Autodesk Inventor part; units mm, degrees
(part 2 of 2)
sketch "Sketch18" plane through (0, 0, 0) normal (0, 0, 1) x (1, 0, 0)
  circle A0 centre (6.1, 11.9) radius 0.15 projected
  circle A1 centre (6.1, 13.5) radius 0.15 projected
  circle A2 centre (22.375, -7.815) radius 0.15 projected
  circle A3 centre (39.71, -9.9) radius 0.15 projected
  circle A4 centre (48.4, -3.8) radius 0.15 projected
  circle A5 centre (55.95, 2.9) radius 0.15 projected
  circle A6 centre (79, 24.8) radius 0.15 projected
  circle A7 centre (52.3, 16.9) radius 0.15 projected
  circle A8 centre (36, 1.1) radius 0.15 projected
  circle A9 centre (83.5, -20.09) radius 0.15 projected
  circle A10 centre (80.4, -15.3) radius 0.15 projected
  circle A11 centre (36.4, -40.4) radius 0.15 projected
  circle A12 centre (17.7, -11.2) radius 0.15 projected
  circle A13 centre (20.6, -14.5) radius 0.15 projected
  circle A14 centre (6.475, -9) radius 0.15 projected
  circle A15 centre (81.1, -6.7) radius 0.15 projected
  circle A16 centre (81.1, -12.3) radius 0.15 projected
  circle A17 centre (67.69, 14.95) radius 0.15 projected
  circle A18 centre (42.638, 24.252) radius 0.15 projected
  circle A19 centre (71.9, 18.8) radius 0.15 projected
  circle A20 centre (42.73, 22.395) radius 0.15 projected
  circle A21 centre (55.56, 27.69) radius 0.15 projected
  circle A22 centre (70.1, 24.7) radius 0.15 projected
  circle A23 centre (82, 18.7) radius 0.15 projected
  circle A24 centre (30.03, 31.595) radius 0.15 projected
  circle A25 centre (29.2, 18.3) radius 0.15 projected
  circle A26 centre (83.6, -26) radius 0.15 projected
  circle A27 centre (83.5, -21.8) radius 0.15 projected
  circle A28 centre (89.2, -12.4) radius 0.15 projected
  circle A29 centre (59.9, -31.6) radius 0.15 projected
  circle A30 centre (36.075, -13.17) radius 0.15 projected
  circle A31 centre (20, -37.1) radius 0.15 projected
  circle A32 centre (9.7, -43.3) radius 0.15 projected
  circle A33 centre (31.7, -33.7) radius 0.15 projected
  circle A34 centre (34.4, -38) radius 0.15 projected
  circle A35 centre (30.5, -43.4) radius 0.15 projected
  circle A36 centre (28.255, -10.955) radius 0.15 projected
  circle A37 centre (28.525, 3.19) radius 0.15 projected
  circle A38 centre (71.4, -31.6) radius 0.15 projected
  circle A39 centre (38.76, -24.905) radius 0.15 projected
  circle A40 centre (64.22, 34.51) radius 0.15 projected
  circle A41 centre (18.46, -4.74) radius 0.15 projected
  circle A42 centre (50.28, 18.42) radius 0.15 projected
  circle A43 centre (22, -40) radius 0.15 projected
  circle A44 centre (27.195, -8.84) radius 0.15 projected
  circle A45 centre (38.3, 36) radius 0.15 projected
  circle A46 centre (74.66, -17.095) radius 0.15 projected
  circle A47 centre (56.99, 5.41) radius 0.15 projected
  circle A48 centre (81.9, 22.5) radius 0.15 projected
  circle A49 centre (25.955, -10.94) radius 0.15 projected
  circle A50 centre (12.3, -10.2) radius 0.15 projected
  circle A51 centre (29.44, -12.665) radius 0.15 projected
  circle A52 centre (26.715, -10.94) radius 0.15 projected
  circle A53 centre (12.3, -9.4) radius 0.15 projected
  circle A54 centre (35.36, -13.43) radius 0.15 projected
  circle A55 centre (26.94, -34.355) radius 0.15 projected
  circle A56 centre (74.56, -18.975) radius 0.15 projected
  circle A57 centre (72.38, 10.4) radius 0.15 projected
  circle A58 centre (28.44, -32.03) radius 0.15 projected
  circle A59 centre (27.66, -34.62) radius 0.15 projected
  circle A60 centre (77.1, -17.9) radius 0.15 projected
  circle A61 centre (76.33, 18.885) radius 0.15 projected
  circle A62 centre (77.1, -18.7) radius 0.15 projected
  circle A63 centre (76.87, 18.35) radius 0.15 projected
  circle A64 centre (27.195, -9.92) radius 0.15 projected
  circle A65 centre (54.885, -4.415) radius 0.15 projected
  circle A66 centre (58.69, -20.96) radius 0.15 projected
  circle A67 centre (30.62, -26.105) radius 0.15 projected
  circle A68 centre (51.44, 19.365) radius 0.15 projected
  circle A69 centre (36.14, 18.41) radius 0.15 projected
  circle A70 centre (58, -20.64) radius 0.15 projected
  circle A71 centre (31.34, -25.84) radius 0.15 projected
  circle A72 centre (50.95, 18.78) radius 0.15 projected
  circle A73 centre (35.36, 18.425) radius 0.15 projected
  circle A74 centre (5.9, -7.5) radius 0.15 projected
  circle A75 centre (27.6, -14.51) radius 0.15 projected
  circle A76 centre (5.9, -10.5) radius 0.15 projected
  circle A77 centre (5.9, -9.5) radius 0.15 projected
  circle A78 centre (18.2, -16.5) radius 0.15 projected
  circle A79 centre (11.9, -15.4) radius 0.15 projected
  circle A80 centre (39.69, 0.21) radius 0.15 projected
  circle A81 centre (30.03, 30.83) radius 0.15 projected
  circle A82 centre (62.6, 19.84) radius 0.15 projected
  circle A83 centre (68.7, 10.4) radius 0.15 projected
  circle A84 centre (48.485, 0.89) radius 0.15 projected
  circle A85 centre (55.7, -14.5) radius 0.15 projected
  circle A86 centre (31.58, -16.8) radius 0.15 projected
  circle A87 centre (60.54, 5.13) radius 0.15 projected
  circle A88 centre (46.6, 2.4) radius 0.15 projected
  circle A89 centre (5.9, 14.5) radius 0.15 projected
  circle A90 centre (27.9, 4.7) radius 0.15 projected
  circle A91 centre (30.67, 6.93) radius 0.15 projected
  circle A92 centre (5.9, 16.5) radius 0.15 projected
  circle A93 centre (27.9, 8.7) radius 0.15 projected
  circle A94 centre (30.67, 8.36) radius 0.15 projected
  circle A95 centre (28.96, 10.535) radius 0.15 projected
  circle A96 centre (5.9, 18.5) radius 0.15 projected
  circle A97 centre (25.9, 15.1) radius 0.15 projected
  circle A98 centre (5.9, 20.5) radius 0.15 projected
  circle A99 centre (27.9, 16.7) radius 0.15 projected
  circle A100 centre (63.455, -20.64) radius 0.15 projected
  circle A101 centre (28.315, -9.36) radius 0.15 projected
  circle A102 centre (18.44, -2.79) radius 0.15 projected
  circle A103 centre (34.67, 7.705) radius 0.15 projected
  circle A104 centre (25.9, 32.7) radius 0.15 projected
  circle A105 centre (29.9, 18) radius 0.15 projected
  circle A106 centre (26.9, 19.2) radius 0.15 projected
  circle A107 centre (27.89, 20.7) radius 0.15 projected
  circle A108 centre (27.8, 23.1) radius 0.15 projected
  circle A109 centre (27.9, 24.7) radius 0.15 projected
  circle A110 centre (28.095, 26.88) radius 0.15 projected
  circle A111 centre (27.9, 28.7) radius 0.15 projected
  circle A112 centre (25.8, 31.1) radius 0.15 projected
  circle A113 centre (25.8, 35.1) radius 0.15 projected
  circle A114 centre (25.9, 36.7) radius 0.15 projected
  circle A115 centre (25.8, 39.1) radius 0.15 projected
  circle A116 centre (27.615, 38.87) radius 0.15 projected
  circle A117 centre (28.03, 40.835) radius 0.15 projected
  circle A118 centre (9.1, 22.5) radius 0.15 projected
  circle A119 centre (9.3, 25.5) radius 0.15 projected
  circle A120 centre (5.9, 26.5) radius 0.15 projected
  circle A121 centre (5.9, 28.5) radius 0.15 projected
  circle A122 centre (5.9, 30.5) radius 0.15 projected
  circle A123 centre (5.9, 32.5) radius 0.15 projected
  circle A124 centre (5.9, 33.5) radius 0.15 projected
  circle A125 centre (5.9, 34.5) radius 0.15 projected
  circle A126 centre (9.55, -9.34) radius 0.15 projected
  circle A127 centre (17.6, -37.7) radius 0.15 projected
  circle A128 centre (30.815, -16.8) radius 0.15 projected
  circle A129 centre (32.1, -44.4) radius 0.15 projected
  circle A130 centre (72.8, 16.2) radius 0.15 projected
  circle A131 centre (30, 39.4) radius 0.15 projected
  circle A132 centre (42.9, -27.9) radius 0.15 projected
  circle A133 centre (45.3, -23.4) radius 0.15 projected
  circle A134 centre (44.5, -24.2) radius 0.15 projected
  circle A135 centre (44.5, -22.6) radius 0.15 projected
  circle A136 centre (19.3, -0.5) radius 0.15 projected
  circle A137 centre (18.5, 0.3) radius 0.15 projected
  circle A138 centre (20.1, 0.3) radius 0.15 projected
  circle A139 centre (19.3, 1.1) radius 0.15 projected
  circle A140 centre (88, -34.7) radius 0.15 projected
  circle A141 centre (43.7, -23.4) radius 0.15 projected
  circle A142 centre (42.3, -22.9) radius 0.15 projected
  circle A143 centre (13, 44.4) radius 0.15 projected
  circle A144 centre (21.8, 36.5) radius 0.15 projected
  circle A145 centre (23.8, 28.5) radius 0.15 projected
  circle A146 centre (23.815, 20.5) radius 0.15 projected
  circle A147 centre (16, 22.5) radius 0.15 projected
  circle A148 centre (14, 30.5) radius 0.15 projected
  circle A149 centre (14, 38.5) radius 0.15 projected
  circle A150 centre (89.2, -34.7) radius 0.15 projected
  circle A151 centre (49.9, -10.235) radius 0.15 projected
  circle A152 centre (38.9, 2.5) radius 0.15 projected
  circle A153 centre (44.92, 10.98) radius 0.15 projected
  circle A154 centre (58.69, 28.175) radius 0.15 projected
  circle A155 centre (37.5, 41.6) radius 0.15 projected
  circle A156 centre (36.7, 43.2) radius 0.15 projected
  circle A157 centre (37.5, 42.4) radius 0.15 projected
  circle A158 centre (21.8, 42) radius 0.15 projected
  circle A159 centre (21.8, 34) radius 0.15 projected
  circle A160 centre (23.9, 22) radius 0.15 projected
  circle A161 centre (16, 23.98) radius 0.15 projected
  circle A162 centre (14.005, 31.98) radius 0.15 projected
  circle A163 centre (14.005, 39.975) radius 0.15 projected
  circle A164 centre (41.7, 39.2) radius 0.15 projected
  circle A165 centre (39.69, -0.55) radius 0.15 projected
  circle A166 centre (79.6, 11.8) radius 0.15 projected
  circle A167 centre (85.6, 12.1) radius 0.15 projected
  circle A168 centre (89.4, -31.4) radius 0.15 projected
  circle A169 centre (17, -12.91) radius 0.15 projected
  circle A170 centre (15.4, -11) radius 0.15 projected
  circle A171 centre (88.2, -12.7) radius 0.15 projected
  circle A172 centre (86.4, -28.8) radius 0.15 projected
  circle A173 centre (81.5, -31.5) radius 0.15 projected
  circle A174 centre (88.4, 13) radius 0.15 projected
  circle A175 centre (85.6, -29.1) radius 0.15 projected
  circle A176 centre (85.2, 28.9) radius 0.15 projected
  circle A177 centre (83, -24.1) radius 0.15 projected
  circle A178 centre (50.4, 11.1) radius 0.15 projected
  circle A179 centre (71.28, -18.24) radius 0.15 projected
  circle A180 centre (61, 18.735) radius 0.15 projected
  circle A181 centre (75.1, 17.3) radius 0.15 projected
  circle A182 centre (46.3, 19.8) radius 0.15 projected
  circle A183 centre (52.5, 14.6) radius 0.15 projected
  circle A184 centre (44.1, 22.1) radius 0.15 projected
  circle A185 centre (36.2, -35.4) radius 0.15 projected
  circle A186 centre (20.9, -41.7) radius 0.15 projected
  circle A187 centre (83.9, -17.2) radius 0.15 projected
  circle A188 centre (34.9, -39.7) radius 0.15 projected
  circle A189 centre (56.315, 27.375) radius 0.15 projected
  circle A190 centre (6.8, -39.2) radius 0.15 projected
  circle A191 centre (73.9, 28.4) radius 0.15 projected
  circle A192 centre (48.3, 26.6) radius 0.15 projected
  circle A193 centre (48.3, 25) radius 0.15 projected
  circle A194 centre (46.7, 25) radius 0.15 projected
  circle A195 centre (23.9, 18) radius 0.15 projected
  circle A196 centre (23.8, 10) radius 0.15 projected
  circle A197 centre (16, 7.98) radius 0.15 projected
  circle A198 centre (16, 15.98) radius 0.15 projected
  circle A199 centre (11.795, 7.67) radius 0.15 projected
  circle A200 centre (52.3, -42.3) radius 0.15 projected
  circle A201 centre (4.3, -36.6) radius 0.15 projected
  circle A202 centre (61, 12.46) radius 0.15 projected
  circle A203 centre (81.5, -26.1) radius 0.15 projected
  circle A204 centre (61.1, -29) radius 0.15 projected
  circle A205 centre (61.9, -29) radius 0.15 projected
  circle A206 centre (62.8, -29.8) radius 0.15 projected
  circle A207 centre (55, -41.1) radius 0.15 projected
  circle A208 centre (55, -40.3) radius 0.15 projected
  circle A209 centre (53, -41.5) radius 0.15 projected
  circle A210 centre (27.1, 15.2) radius 0.15 projected
  circle A211 centre (23.8, 12.5) radius 0.15 projected
  circle A212 centre (23.8, 4.5) radius 0.15 projected
  circle A213 centre (16, 10.5) radius 0.15 projected
  circle A214 centre (20.7, -36.8) radius 0.15 projected
  circle A215 centre (55.96, 26.7) radius 0.15 projected
  circle A216 centre (28.4, -18.5) radius 0.15 projected
  circle A217 centre (44.5, -14.6) radius 0.15 projected
  circle A218 centre (50.3, 2) radius 0.15 projected
  circle A219 centre (46.1, -10.8) radius 0.15 projected
  circle A220 centre (51.395, 20.445) radius 0.15 projected
  circle A221 centre (77.6, 23.5) radius 0.15 projected
  circle A222 centre (36.1, 2.8) radius 0.15 projected
  circle A223 centre (61.465, -22.4) radius 0.15 projected
  circle A224 centre (80.3, -11.5) radius 0.15 projected
  circle A225 centre (80.1, -35.8) radius 0.15 projected
  circle A226 centre (29.2, -42.7) radius 0.15 projected
  circle A227 centre (36.025, 15.595) radius 0.15 projected
  circle A228 centre (29.8, 34.1) radius 0.15 projected
  circle A229 centre (22.4, -12.1) radius 0.15 projected
  circle A230 centre (8.09, -8.99) radius 0.15 projected
  circle A231 centre (72.62, -11.01) radius 0.15 projected
  circle A232 centre (66.42, 15.715) radius 0.15 projected
  circle A233 centre (53.89, -5.83) radius 0.15 projected
  circle A234 centre (72.94, -11.7) radius 0.15 projected
  circle A235 centre (69.5, 19.215) radius 0.15 projected
  circle A236 centre (71.76, -12.19) radius 0.15 projected
  circle A237 centre (65.88, 16.255) radius 0.15 projected
  circle A238 centre (53.71, -6.57) radius 0.15 projected
  circle A239 centre (58.84, -22.08) radius 0.15 projected
  circle A240 centre (67.3, 19.215) radius 0.15 projected
  circle A241 centre (81.7, -33.4) radius 0.15 projected
  circle A242 centre (5.3, -38.3) radius 0.15 projected
  circle A243 centre (83.355, -3.96) radius 0.15 projected
  circle A244 centre (84.5, 13.8) radius 0.15 projected
  circle A245 centre (82.7, -14.2) radius 0.15 projected
  circle A246 centre (83.5, -14.2) radius 0.15 projected
  circle A247 centre (83.5, -15) radius 0.15 projected
  circle A248 centre (82.7, -15.8) radius 0.15 projected
  circle A249 centre (66.3, -36.73) radius 0.15 projected
  circle A250 centre (68.5, 37.65) radius 0.15 projected
  circle A251 centre (70.2, -37.9) radius 0.15 projected
  circle A252 centre (37.8, -35.6) radius 0.15 projected
  circle A253 centre (38.7, -41.5) radius 0.15 projected
  circle A254 centre (38.7, -35.5) radius 0.15 projected
  circle A255 centre (72, 27.6) radius 0.15 projected
  circle A256 centre (71.18, 27.71) radius 0.15 projected
  circle A257 centre (69, 28.1) radius 0.15 projected
  circle A258 centre (56.4, 36.81) radius 0.15 projected
  circle A259 centre (81.5, 14.6) radius 0.15 projected
  circle A260 centre (82.1, 15.2) radius 0.15 projected
  circle A261 centre (81.8, 17.59) radius 0.15 projected
  circle A262 centre (81.2, 16.99) radius 0.15 projected
  circle A263 centre (81.5, 15.2) radius 0.15 projected
  circle A264 centre (62.8, -39.2) radius 0.15 projected
  circle A265 centre (71.39, -36.73) radius 0.15 projected
  circle A266 centre (62, 39.1) radius 0.15 projected
  circle A267 centre (70, 28.3) radius 0.15 projected
  circle A268 centre (69.9, -2.2) radius 0.15 projected
  circle A269 centre (81.78, -23.295) radius 0.15 projected
  circle A270 centre (72.04, -18.24) radius 0.15 projected
  circle A271 centre (71.4, -7.4) radius 0.15 projected
  circle A272 centre (87.095, 35.64) radius 0.15 projected
  circle A273 centre (72.76, -19.96) radius 0.15 projected
  circle A274 centre (85.155, -30.25) radius 0.15 projected
  circle A275 centre (77.34, 13.12) radius 0.15 projected
  circle A276 centre (78.29, -34.2) radius 0.15 projected
  circle A277 centre (6.1, 6.3) radius 0.15 projected
  circle A278 centre (6.1, 7.9) radius 0.15 projected
  circle A279 centre (6.1, 9.5) radius 0.15 projected
  circle A280 centre (6.1, 11.1) radius 0.15 projected
  circle A281 centre (41, -36.2) radius 0.15 projected
  circle A282 centre (45.6, 19.5) radius 0.15 projected
  circle A283 centre (35.7, -24.95) radius 0.15 projected
  circle A284 centre (82, 13.8) radius 0.15 projected
  circle A285 centre (83.2, 10.9) radius 0.15 projected
  circle A286 centre (43.2, 20.1) radius 0.15 projected
  circle A287 centre (77.9, 41.2) radius 0.15 projected
  circle A288 centre (89.4, -37.7) radius 0.15 projected
  circle A289 centre (59.1, -32.9) radius 0.15 projected
  circle A290 centre (79.8, -31.7) radius 0.15 projected
  circle A291 centre (12, -41.3) radius 0.15 projected
  circle A292 centre (70.1, -34.7) radius 0.15 projected
  circle A293 centre (68.2, -38.9) radius 0.15 projected
  circle A294 centre (73.8, -42.9) radius 0.15 projected
  circle A295 centre (64.8, -42.9) radius 0.15 projected
  circle A296 centre (53.1, -31.5) radius 0.15 projected
  circle A297 centre (52.6, -28) radius 0.15 projected
  circle A298 centre (51.8, -28.8) radius 0.15 projected
  circle A299 centre (50.2, -28.8) radius 0.15 projected
  circle A300 centre (42.4, -37.1) radius 0.15 projected
  circle A301 centre (42.4, -35.4) radius 0.15 projected
  circle A302 centre (42.2, -39.8) radius 0.15 projected
  circle A303 centre (41, -39.8) radius 0.15 projected
  circle A304 centre (41, -37.8) radius 0.15 projected
  circle A305 centre (42.2, -37.8) radius 0.15 projected
  circle A306 centre (47.4, -43) radius 0.15 projected
  circle A307 centre (47.4, -44.4) radius 0.15 projected
  circle A308 centre (46.6, -43.1) radius 0.15 projected
  circle A309 centre (35.3, 27.2) radius 0.15 projected
  circle A310 centre (29.47, 15.2) radius 0.15 projected
  circle A311 centre (22, 18.695) radius 0.15 projected
  circle A312 centre (69.7, 29.7) radius 0.15 projected
  circle A313 centre (64.2, 32.9) radius 0.15 projected
  circle A314 centre (73.5, 33) radius 0.15 projected
  circle A315 centre (68.2, 36.7) radius 0.15 projected
  circle A316 centre (61.95, 43.2) radius 0.15 projected
  circle A317 centre (57.2, 38.9) radius 0.15 projected
  circle A318 centre (40.5, 30) radius 0.15 projected
  circle A319 centre (44, 19.5) radius 0.15 projected
  circle A320 centre (43.2, 20.7) radius 0.15 projected
  circle A321 centre (39.8, 35.2) radius 0.15 projected
  circle A322 centre (39.8, 36.4) radius 0.15 projected
  circle A323 centre (41.8, 36.4) radius 0.15 projected
  circle A324 centre (41.8, 35.2) radius 0.15 projected
  circle A325 centre (39.7, 31.6) radius 0.15 projected
  circle A326 centre (36.9, 39.6) radius 0.15 projected
  circle A327 centre (35.2, 38.8) radius 0.15 projected
  circle A328 centre (35.2, 40.4) radius 0.15 projected
  circle A329 centre (51.4, 42.2) radius 0.15 projected
  circle A330 centre (51.4, 43.8) radius 0.15 projected
  circle A331 centre (52.5, 35.9) radius 0.15 projected
  circle A332 centre (12.8, -10.8) radius 0.15 projected
  circle A333 centre (21.7, 39.7) radius 0.15 projected
  circle A334 centre (21.69, 31.695) radius 0.15 projected
  circle A335 centre (23.7, 23.7) radius 0.15 projected
  circle A336 centre (23.7, 15.7) radius 0.15 projected
  circle A337 centre (23.7, 7.7) radius 0.15 projected
  circle A338 centre (15.9, 5.7) radius 0.15 projected
  circle A339 centre (15.9, 13.7) radius 0.15 projected
  circle A340 centre (16, 21.7) radius 0.15 projected
  circle A341 centre (13.9, 29.7) radius 0.15 projected
  circle A342 centre (13.9, 41.7) radius 0.15 projected
  circle A343 centre (13.9, 37.7) radius 0.15 projected
  circle A344 centre (13.9, 33.7) radius 0.15 projected
  circle A345 centre (16, 25.7) radius 0.15 projected
  circle A346 centre (16, 17.7) radius 0.15 projected
  circle A347 centre (16, 9.7) radius 0.15 projected
  circle A348 centre (23.7, 3.7) radius 0.15 projected
  circle A349 centre (23.915, 11.745) radius 0.15 projected
  circle A350 centre (23.765, 19.74) radius 0.15 projected
  circle A351 centre (23.7, 27.7) radius 0.15 projected
  circle A352 centre (21.7, 35.7) radius 0.15 projected
  circle A353 centre (10.29, 10.02) radius 0.15 projected
  circle A354 centre (37.7, 36.5) radius 0.15 projected
  circle A355 centre (51.3, 31.8) radius 0.15 projected
  circle A356 centre (51.4, 43) radius 0.15 projected
  circle A357 centre (52.2, 42.2) radius 0.15 projected
  circle A358 centre (35.2, 39.6) radius 0.15 projected
  circle A359 centre (36.9, 40.4) radius 0.15 projected
  circle A360 centre (36.9, 38.8) radius 0.15 projected
  circle A361 centre (39.7, 30.8) radius 0.15 projected
  circle A362 centre (42.1, 35.8) radius 0.15 projected
  circle A363 centre (40.8, 36.5) radius 0.15 projected
  circle A364 centre (39.5, 35.8) radius 0.15 projected
  circle A365 centre (43.2, 19.5) radius 0.15 projected
  circle A366 centre (44.8, 19.5) radius 0.15 projected
  circle A367 centre (40.5, 31.6) radius 0.15 projected
  circle A368 centre (57.2, 36) radius 0.15 projected
  circle A369 centre (64.8, 40.7) radius 0.15 projected
  circle A370 centre (59.3, 30.1) radius 0.15 projected
  circle A371 centre (71, 36.7) radius 0.15 projected
  circle A372 centre (63.6, 30.8) radius 0.15 projected
  circle A373 centre (66.6, 31.9) radius 0.15 projected
  circle A374 centre (10.6, 42) radius 0.15 projected
  circle A375 centre (22, 9.7) radius 0.15 projected
  circle A376 centre (40, 22.6) radius 0.15 projected
  circle A377 centre (39.4, 27.1) radius 0.15 projected
  circle A378 centre (46.6, -44.4) radius 0.15 projected
  circle A379 centre (47.4, -43.7) radius 0.15 projected
  circle A380 centre (46.6, -43.7) radius 0.15 projected
  circle A381 centre (41.6, -37.8) radius 0.15 projected
  circle A382 centre (40.9, -38.8) radius 0.15 projected
  circle A383 centre (41.6, -40.1) radius 0.15 projected
  circle A384 centre (41.6, -35.4) radius 0.15 projected
  circle A385 centre (43.2, -35.4) radius 0.15 projected
  circle A386 centre (41.7, -37.1) radius 0.15 projected
  circle A387 centre (51, -28.8) radius 0.15 projected
  circle A388 centre (52.6, -28.8) radius 0.15 projected
  circle A389 centre (52.6, -27.2) radius 0.15 projected
  circle A390 centre (57.6, -40) radius 0.15 projected
  circle A391 centre (64.7, -39.8) radius 0.15 projected
  circle A392 centre (73.5, -40.62) radius 0.15 projected
  circle A393 centre (64.7, -34.7) radius 0.15 projected
  circle A394 centre (60, -34.6) radius 0.15 projected
  circle A395 centre (6.7, -40.65) radius 0.15 projected
  circle A396 centre (84.6, -33) radius 0.15 projected
  circle A397 centre (82.75, -5.8) radius 0.15 projected
  circle A398 centre (54, 33) radius 0.15 projected
  circle A399 centre (77.7, 35) radius 0.15 projected
  circle A400 centre (45.6, 20.1) radius 0.15 projected
  circle A401 centre (78.415, 10.635) radius 0.15 projected
  circle A402 centre (58, 1.5) radius 0.15 projected
  circle A403 centre (38.2, -15.4) radius 0.15 projected
  circle A404 centre (52.2, 43) radius 0.15 projected
  circle A405 centre (41, -37) radius 0.15 projected
  circle A406 centre (6.1, 10.3) radius 0.15 projected
  circle A407 centre (6.1, 8.7) radius 0.15 projected
  circle A408 centre (6.1, 7.1) radius 0.15 projected
  circle A409 centre (6.1, 5.5) radius 0.15 projected
  circle A410 centre (87.1, 36.4) radius 0.15 projected
  circle A411 centre (71.66, -8.115) radius 0.15 projected
  circle A412 centre (72.8, -18.24) radius 0.15 projected
  circle A413 centre (78.29, -35) radius 0.15 projected
  circle A414 centre (77.335, 13.88) radius 0.15 projected
  circle A415 centre (85.155, -31.015) radius 0.15 projected
  circle A416 centre (72, -19.96) radius 0.15 projected
  circle A417 centre (66, -2.185) radius 0.15 projected
  circle A418 centre (56.6, 33.9) radius 0.15 projected
  circle A419 centre (68.4, 33.9) radius 0.15 projected
  circle A420 centre (60.9, 32.5) radius 0.15 projected
  circle A421 centre (62.5, -35.8) radius 0.15 projected
  circle A422 centre (67.1, -32.9) radius 0.15 projected
  circle A423 centre (81.8, 16.99) radius 0.15 projected
  circle A424 centre (80.6, 16.99) radius 0.15 projected
  circle A425 centre (81.2, 17.59) radius 0.15 projected
  circle A426 centre (82.1, 14.6) radius 0.15 projected
  circle A427 centre (68.2, 2) radius 0.15 projected
  circle A428 centre (62, 33.1) radius 0.15 projected
  circle A429 centre (74.5, 37.3) radius 0.15 projected
  circle A430 centre (72.5, 34.9) radius 0.15 projected
  circle A431 centre (58, -36.75) radius 0.15 projected
  circle A432 centre (59.1, -39.8) radius 0.15 projected
  circle A433 centre (75, -37.9) radius 0.15 projected
  circle A434 centre (75.5, -41.6) radius 0.15 projected
  circle A435 centre (37.86, -38.715) radius 0.15 projected
  circle A436 centre (66.3, -43.2) radius 0.15 projected
  circle A437 centre (84.3, -15) radius 0.15 projected
  circle A438 centre (83.5, -15.8) radius 0.15 projected
  circle A439 centre (84.3, -14.2) radius 0.15 projected
  circle A440 centre (82.7, -15) radius 0.15 projected
  circle A441 centre (65.6, 33.5) radius 0.15 projected
  circle A442 centre (70.7, -4.8) radius 0.15 projected
  circle A443 centre (77, 37.5) radius 0.15 projected
  circle A444 centre (18.7, -43.7) radius 0.15 projected
  circle A445 centre (87.2, -34.6) radius 0.15 projected
  circle A446 centre (65.34, 16.795) radius 0.15 projected
  circle A447 centre (71.54, -11.46) radius 0.15 projected
  circle A448 centre (68, 18.915) radius 0.15 projected
  circle A449 centre (58.08, -22.08) radius 0.15 projected
  circle A450 centre (54.345, -6.99) radius 0.15 projected
  circle A451 centre (66.96, 15.175) radius 0.15 projected
  circle A452 centre (59.17, -23.16) radius 0.15 projected
  circle A453 centre (68.8, 18.915) radius 0.15 projected
  circle A454 centre (59.93, -23.17) radius 0.15 projected
  circle A455 centre (54.57, -5.49) radius 0.15 projected
  circle A456 centre (6.2, -11.2) radius 0.15 projected
  circle A457 centre (22.4, -15) radius 0.15 projected
  circle A458 centre (34.9, 32.9) radius 0.15 projected
  circle A459 centre (28.5, -39.9) radius 0.15 projected
  circle A460 centre (13.9, -44) radius 0.15 projected
  circle A461 centre (77.395, -37.24) radius 0.15 projected
  circle A462 centre (78.1, -11.1) radius 0.15 projected
  circle A463 centre (47.7, 6.3) radius 0.15 projected
  circle A464 centre (22.6, -0.4) radius 0.15 projected
  circle A465 centre (63.7, 13.27) radius 0.15 projected
  circle A466 centre (44.8, 13.3) radius 0.15 projected
  circle A467 centre (38.1, -9.9) radius 0.15 projected
  circle A468 centre (61.82, -4.17) radius 0.15 projected
  circle A469 centre (24.9, -17.7) radius 0.15 projected
  circle A470 centre (64.69, 33.91) radius 0.15 projected
  circle A471 centre (39.3, -25.44) radius 0.15 projected
  circle A472 centre (16, 14.5) radius 0.15 projected
  circle A473 centre (16, 6.5) radius 0.15 projected
  circle A474 centre (23.8, 8.5) radius 0.15 projected
  circle A475 centre (23.8, 16.5) radius 0.15 projected
  circle A476 centre (52.3, -41.5) radius 0.15 projected
  circle A477 centre (53, -42.3) radius 0.15 projected
  circle A478 centre (55.8, -40.3) radius 0.15 projected
  circle A479 centre (62.8, -29) radius 0.15 projected
  circle A480 centre (61.9, -29.8) radius 0.15 projected
  circle A481 centre (61.9, -28.2) radius 0.15 projected
  circle A482 centre (61.1, -28.2) radius 0.15 projected
  circle A483 centre (81.2, 25.9) radius 0.15 projected
  circle A484 centre (51.3, -13.2) radius 0.15 projected
  circle A485 centre (61.1, -29.8) radius 0.15 projected
  circle A486 centre (53.8, -42.3) radius 0.15 projected
  circle A487 centre (12.3, 7.1) radius 0.15 projected
  circle A488 centre (15.995, 11.98) radius 0.15 projected
  circle A489 centre (23.8, 6) radius 0.15 projected
  circle A490 centre (23.8, 14) radius 0.15 projected
  circle A491 centre (45.9, 25) radius 0.15 projected
  circle A492 centre (47.5, 25) radius 0.15 projected
  circle A493 centre (48.3, 25.8) radius 0.15 projected
  circle A494 centre (82, -4.3) radius 0.15 projected
  circle A495 centre (64.22, 18.4) radius 0.15 projected
  circle A496 centre (13.7, 4.4) radius 0.15 projected
  circle A497 centre (40.7, -42.7) radius 0.15 projected
  circle A498 centre (83.9, -22.5) radius 0.15 projected
  circle A499 centre (82.4, -25.6) radius 0.15 projected
  circle A500 centre (24, -42.8) radius 0.15 projected
  circle A501 centre (81.9, 23.3) radius 0.15 projected
  circle A502 centre (54.4, 15.9) radius 0.15 projected
  circle A503 centre (26.7, -4.3) radius 0.15 projected
  circle A504 centre (71.18, 17.96) radius 0.15 projected
  circle A505 centre (71.66, 12.95) radius 0.15 projected
  circle A506 centre (65.465, 13.585) radius 0.15 projected
  circle A507 centre (36, 4.7) radius 0.15 projected
  circle A508 centre (89.8, 14.2) radius 0.15 projected
  circle A509 centre (82.2, -24.1) radius 0.15 projected
  circle A510 centre (84.4, 28.9) radius 0.15 projected
  circle A511 centre (88.6, 28.4) radius 0.15 projected
  circle A512 centre (81, 31.3) radius 0.15 projected
  circle A513 centre (87.2, -28.8) radius 0.15 projected
  circle A514 centre (88.3, -31.1) radius 0.15 projected
  circle A515 centre (87.4, -12.7) radius 0.15 projected
  circle A516 centre (15.4, -12.6) radius 0.15 projected
  circle A517 centre (15.45, -35.315) radius 0.15 projected
  circle A518 centre (87.3, 12.1) radius 0.15 projected
  circle A519 centre (69.8, 2.8) radius 0.15 projected
  circle A520 centre (5.9, -5.5) radius 0.15 projected
  circle A521 centre (78.82, 13.46) radius 0.15 projected
  circle A522 centre (14, 44) radius 0.15 projected
  circle A523 centre (14, 35.98) radius 0.15 projected
  circle A524 centre (16.005, 27.98) radius 0.15 projected
  circle A525 centre (16, 19.98) radius 0.15 projected
  circle A526 centre (23.8, 26) radius 0.15 projected
  circle A527 centre (21.8, 38) radius 0.15 projected
  circle A528 centre (23.58, 30.6) radius 0.15 projected
  circle A529 centre (36.7, 42.4) radius 0.15 projected
  circle A530 centre (37.5, 43.2) radius 0.15 projected
  circle A531 centre (36.7, 41.6) radius 0.15 projected
  circle A532 centre (48.935, 19.86) radius 0.15 projected
  circle A533 centre (57.11, -21.28) radius 0.15 projected
  circle A534 centre (38.9, 4.2) radius 0.15 projected
  circle A535 centre (83, -37) radius 0.15 projected
  circle A536 centre (14, 42.5) radius 0.15 projected
  circle A537 centre (14, 34.5) radius 0.15 projected
  circle A538 centre (16, 26.5) radius 0.15 projected
  circle A539 centre (16, 18.5) radius 0.15 projected
  circle A540 centre (23.8, 24.5) radius 0.15 projected
  circle A541 centre (21.765, 32.54) radius 0.15 projected
  circle A542 centre (21.8, 40.5) radius 0.15 projected
  circle A543 centre (42.9, -22.6) radius 0.15 projected
  circle A544 centre (43.7, -22.6) radius 0.15 projected
  circle A545 centre (43.7, -24.2) radius 0.15 projected
  circle A546 centre (18.5, 1.1) radius 0.15 projected
  circle A547 centre (20.1, 1.1) radius 0.15 projected
  circle A548 centre (19.3, 0.3) radius 0.15 projected
  circle A549 centre (18.5, -0.5) radius 0.15 projected
  circle A550 centre (42.295, -15.04) radius 0.15 projected
  circle A551 centre (44.5, -23.4) radius 0.15 projected
  circle A552 centre (45.3, -24.2) radius 0.15 projected
  circle A553 centre (45.3, -22.6) radius 0.15 projected
  circle A554 centre (39.9, -33.9) radius 0.15 projected
  circle A555 centre (74.765, 16.16) radius 0.15 projected
  circle A556 centre (39.2, -44) radius 0.15 projected
  circle A557 centre (28.855, -9.895) radius 0.15 projected
  circle A558 centre (39.98, -26.8) radius 0.15 projected
  circle A559 centre (5.9, 35.5) radius 0.15 projected
  circle A560 centre (10.1, -6.5) radius 0.15 projected
  circle A561 centre (12.1, 40.835) radius 0.15 projected
  circle A562 centre (11.7, 39.45) radius 0.15 projected
  circle A563 centre (5.9, 31.5) radius 0.15 projected
  circle A564 centre (5.9, 29.5) radius 0.15 projected
  circle A565 centre (5.9, 27.5) radius 0.15 projected
  circle A566 centre (5.9, 25.6) radius 0.15 projected
  circle A567 centre (5.9, 22.4) radius 0.15 projected
  circle A568 centre (5.9, 21.5) radius 0.15 projected
  circle A569 centre (33.84, 20.76) radius 0.15 projected
  circle A570 centre (33.67, 20.015) radius 0.15 projected
  circle A571 centre (32.76, 20.76) radius 0.15 projected
  circle A572 centre (32, 20.76) radius 0.15 projected
  circle A573 centre (31.87, 20.01) radius 0.15 projected
  circle A574 centre (32.37, 17.98) radius 0.15 projected
  circle A575 centre (32.19, 15.57) radius 0.15 projected
  circle A576 centre (32.49, 14.87) radius 0.15 projected
  circle A577 centre (32.01, 14.28) radius 0.15 projected
  circle A578 centre (33.8, 9.5) radius 0.15 projected
  circle A579 centre (30.03, 12.85) radius 0.15 projected
  circle A580 centre (33.165, 9.08) radius 0.15 projected
  circle A581 centre (41.53, 21.79) radius 0.15 projected
  circle A582 centre (31.87, 19.245) radius 0.15 projected
  circle A583 centre (29.71, 3.92) radius 0.15 projected
  circle A584 centre (20.29, -10.94) radius 0.15 projected
  circle A585 centre (31.88, -25.3) radius 0.15 projected
  circle A586 centre (46.1, -6.8) radius 0.15 projected
  circle A587 centre (29.71, 11.64) radius 0.15 projected
  circle A588 centre (5.9, 19.5) radius 0.15 projected
  circle A589 centre (29.68, 10.88) radius 0.15 projected
  circle A590 centre (27.89, 12.5) radius 0.15 projected
  circle A591 centre (28.2, 10.6) radius 0.15 projected
  circle A592 centre (34.8, -43.4) radius 0.15 projected
  circle A593 centre (30.93, 7.645) radius 0.15 projected
  circle A594 centre (27.8, 7.3) radius 0.15 projected
  circle A595 centre (5.9, 15.5) radius 0.15 projected
  circle A596 centre (45.85, 4.725) radius 0.15 projected
  circle A597 centre (60, 3.5) radius 0.15 projected
  circle A598 centre (31.03, 2.045) radius 0.15 projected
  circle A599 centre (29.395, -9.36) radius 0.15 projected
  circle A600 centre (55.7, -15.63) radius 0.15 projected
  circle A601 centre (81.79, 24.055) radius 0.15 projected
  circle A602 centre (66.69, 5.48) radius 0.15 projected
  circle A603 centre (81.9, 26.3) radius 0.15 projected
  circle A604 centre (28.7, 39.8) radius 0.15 projected
  circle A605 centre (40.01, 0.9) radius 0.15 projected
  circle A606 centre (41.41, 0.69) radius 0.15 projected
  circle A607 centre (18.7, -10.605) radius 0.15 projected
  circle A608 centre (18.7, -14.1) radius 0.15 projected
  circle A609 centre (5.9, -8.5) radius 0.15 projected
  circle A610 centre (41.09, 0) radius 0.15 projected
  circle A611 centre (24.875, -10.94) radius 0.15 projected
  circle A612 centre (33.9, 32.1) radius 0.15 projected
  circle A613 centre (15.01, -42.2) radius 0.15 projected
  circle A614 centre (19.26, -3.56) radius 0.15 projected
  circle A615 centre (51.675, -11.495) radius 0.15 projected
  circle A616 centre (34.66, 32.175) radius 0.15 projected
  circle A617 centre (15.21, -43.025) radius 0.15 projected
  circle A618 centre (19.525, -4.275) radius 0.15 projected
  circle A619 centre (52.215, -10.96) radius 0.15 projected
  circle A620 centre (48.5, -1.81) radius 0.15 projected
  circle A621 centre (12.3, -7.8) radius 0.15 projected
  circle A622 centre (28.285, -14.12) radius 0.15 projected
  circle A623 centre (71.62, 10.405) radius 0.15 projected
  circle A624 centre (74.02, -18.435) radius 0.15 projected
  circle A625 centre (71.62, 9.63) radius 0.15 projected
  circle A626 centre (73.48, -17.9) radius 0.15 projected
  circle A627 centre (28.44, -33.87) radius 0.15 projected
  circle A628 centre (77.41, 18.885) radius 0.15 projected
  circle A629 centre (77.1, -19.5) radius 0.15 projected
  circle A630 centre (28.12, -33.18) radius 0.15 projected
  circle A631 centre (50.5, 7.1) radius 0.15 projected
  circle A632 centre (16.1, -35.72) radius 0.15 projected
  circle A633 centre (28.9, -13.205) radius 0.15 projected
  circle A634 centre (12.3, -8.6) radius 0.15 projected
  circle A635 centre (27.475, -10.94) radius 0.15 projected
  circle A636 centre (29.44, -13.745) radius 0.15 projected
  circle A637 centre (36.65, -41.35) radius 0.15 projected
  circle A638 centre (77.95, 18.35) radius 0.15 projected
  circle A639 centre (5.9, 17.5) radius 0.15 projected
  circle A640 centre (48.4, -3) radius 0.15 projected
  circle A641 centre (40.95, 23.5) radius 0.15 projected
  circle A642 centre (57.3, 13.8) radius 0.15 projected
  circle A643 centre (61.67, 19.095) radius 0.15 projected
  circle A644 centre (25.2, -38.3) radius 0.15 projected
  circle A645 centre (14.2, -34.58) radius 0.15 projected
  circle A646 centre (56.72, 26.73) radius 0.15 projected
  circle A647 centre (14.96, -35.9) radius 0.15 projected
  circle A648 centre (63.735, -31.04) radius 0.15 projected
  circle A649 centre (40.1, -20.565) radius 0.15 projected
  circle A650 centre (87.7, -33.2) radius 0.15 projected
  circle A651 centre (40.7, -44) radius 0.15 projected
  circle A652 centre (34.5, -35.8) radius 0.15 projected
  circle A653 centre (22.1, -43.9) radius 0.15 projected
  circle A654 centre (39.66, -26.11) radius 0.15 projected
  circle A655 centre (18.72, -5.455) radius 0.15 projected
  circle A656 centre (70.6, -31.6) radius 0.15 projected
  circle A657 centre (86, -12.4) radius 0.15 projected
  circle A658 centre (78.9, -21.3) radius 0.15 projected
  circle A659 centre (81.4, -22.6) radius 0.15 projected
  circle A660 centre (84.8, -29.1) radius 0.15 projected
  circle A661 centre (29.2, 39.2) radius 0.15 projected
  circle A662 centre (63.68, 35.415) radius 0.15 projected
  circle A663 centre (78.71, 18.4) radius 0.15 projected
  circle A664 centre (73, 21.9) radius 0.15 projected
  circle A665 centre (57.5, 16) radius 0.15 projected
  circle A666 centre (29.6, -4.4) radius 0.15 projected
  circle A667 centre (71.79, 13.7) radius 0.15 projected
  circle A668 centre (55.9, 13.9) radius 0.15 projected
  circle A669 centre (88.44, 15.85) radius 0.15 projected
  circle A670 centre (78.18, -10.195) radius 0.15 projected
  circle A671 centre (71.46, -20.495) radius 0.15 projected
  circle A672 centre (6.475, -7) radius 0.15 projected
  circle A673 centre (20.6, -17.3) radius 0.15 projected
  circle A674 centre (31.1, 33.25) radius 0.15 projected
  circle A675 centre (29.4, -39.5) radius 0.15 projected
  circle A676 centre (80.1, -33.8) radius 0.15 projected
  circle A677 centre (46.9, 6.3) radius 0.15 projected
  circle A678 centre (23.9, -1.6) radius 0.15 projected
  circle A679 centre (37.1, 16.6) radius 0.15 projected
  circle A680 centre (21.1, -42.5) radius 0.15 projected
  circle A681 centre (57, -2.2) radius 0.15 projected
  circle A682 centre (47.5, -10.8) radius 0.15 projected
  circle A683 centre (54, 5.6) radius 0.15 projected
  circle A684 centre (53.9, 1) radius 0.15 projected
  circle A685 centre (6.1, 12.7) radius 0.15 projected
  circle A686 centre (82.985, -17.14) radius 0.15 projected
  circle A687 centre (58.9, -42.5) radius 0.175 projected
  circle A688 centre (37.4, -31.2) radius 0.175 projected
  circle A689 centre (35.8, -29.6) radius 0.175 projected
  circle A690 centre (57.3, 44.1) radius 0.175 projected
  circle A691 centre (38.531, 28.469) radius 0.175 projected
  circle A692 centre (56.169, 41.369) radius 0.175 projected
  circle A693 centre (56.169, 43.631) radius 0.175 projected
  circle A694 centre (58.431, 43.631) radius 0.175 projected
  circle A695 centre (88.531, -4.369) radius 0.175 projected
  circle A696 centre (37.4, 28) radius 0.175 projected
  circle A697 centre (35.8, 29.6) radius 0.175 projected
  circle A698 centre (37.4, 31.2) radius 0.175 projected
  circle A699 centre (39, 29.6) radius 0.175 projected
  circle A700 centre (88.531, -6.631) radius 0.175 projected
  circle A701 centre (86.269, -6.631) radius 0.175 projected
  circle A702 centre (86.269, -4.369) radius 0.175 projected
  circle A703 centre (77.031, 4.369) radius 0.175 projected
  circle A704 centre (74.769, 4.369) radius 0.175 projected
  circle A705 centre (74.769, 6.631) radius 0.175 projected
  circle A706 centre (77.031, 6.631) radius 0.175 projected
  circle A707 centre (58.431, -43.631) radius 0.175 projected
  circle A708 centre (56.169, -43.631) radius 0.175 projected
  circle A709 centre (56.169, -41.369) radius 0.175 projected
  circle A710 centre (58.431, -41.369) radius 0.175 projected
  circle A711 centre (57.3, -40.9) radius 0.175 projected
  circle A712 centre (55.7, -42.5) radius 0.175 projected
  circle A713 centre (57.3, -44.1) radius 0.175 projected
  circle A714 centre (77.5, 5.5) radius 0.175 projected
  circle A715 centre (75.9, 7.1) radius 0.175 projected
  circle A716 centre (74.3, 5.5) radius 0.175 projected
  circle A717 centre (75.9, 3.9) radius 0.175 projected
  circle A718 centre (87.4, -3.9) radius 0.175 projected
  circle A719 centre (85.8, -5.5) radius 0.175 projected
  circle A720 centre (87.4, -7.1) radius 0.175 projected
  circle A721 centre (89, -5.5) radius 0.175 projected
  circle A722 centre (38.531, 30.731) radius 0.175 projected
  circle A723 centre (36.269, 30.731) radius 0.175 projected
  circle A724 centre (36.269, 28.469) radius 0.175 projected
  circle A725 centre (39, -29.6) radius 0.175 projected
  circle A726 centre (58.9, 42.5) radius 0.175 projected
  circle A727 centre (38.531, -28.469) radius 0.175 projected
  circle A728 centre (55.7, 42.5) radius 0.175 projected
  circle A729 centre (57.3, 40.9) radius 0.175 projected
  circle A730 centre (37.4, -28) radius 0.175 projected
  circle A731 centre (36.269, -28.469) radius 0.175 projected
  circle A732 centre (36.269, -30.731) radius 0.175 projected
  circle A733 centre (38.531, -30.731) radius 0.175 projected
  circle A734 centre (58.431, 41.369) radius 0.175 projected
  circle A735 centre (34.1, 39.2) radius 0.35 projected
  circle A736 centre (87.975, 4.15) radius 0.35 projected
  circle A737 centre (80.725, 4.15) radius 0.35 projected
  circle A738 centre (36.1, -33.4) radius 0.35 projected
  circle A739 centre (7.9, 9.6) radius 0.5 projected
  circle A740 centre (12.3, -3.9) radius 0.5 projected
  circle A741 centre (62.54, -8) radius 0.6 projected
  circle A742 centre (62.54, 8) radius 0.6 projected
  circle A743 centre (57.46, 8) radius 0.6 projected
  circle A744 centre (57.46, -8) radius 0.6 projected
  circle A745 centre (37.4, 29.6) radius 1.1 projected
  circle A746 centre (87.4, -5.5) radius 1.1 projected
  circle A747 centre (37.4, -29.6) radius 1.1 projected
  circle A748 centre (57.3, -42.5) radius 1.1 projected
  circle A749 centre (75.9, 5.5) radius 1.1 projected
  circle A750 centre (57.3, 42.5) radius 1.1 projected
  circle A751 centre (32.5, -11.5) radius 1.5 projected
  circle A752 centre (32.5, 11.5) radius 1.5 projected
  circle A753 centre (76, 30.5) radius 1.5 projected
  circle A754 centre (76, -30.5) radius 1.5 projected
  circle A755 centre (32.5, 30.5) radius 1.5 projected
  circle A756 centre (76, 11.5) radius 1.5 projected
  circle A757 centre (76, -11.5) radius 1.5 projected
  circle A758 centre (32.5, -30.5) radius 1.5 projected
  arc A759 (90.4, 34) -> (89.4, 35) centre (89.4, 34) ccw projected
  arc A760 (88.4, 36) -> (89.4, 35) centre (89.4, 36) ccw projected
  line L0 (88.4, 36) -> (88.4, 42) projected
  arc A761 (89.4, 43) -> (88.4, 42) centre (89.4, 42) ccw projected
  arc A762 (89.4, 43) -> (90.4, 44) centre (89.4, 44) ccw projected
  line L1 (90.4, 44) -> (90.4, 47.4) projected
  arc A763 (90.4, 47.4) -> (89.9, 47.9) centre (89.9, 47.4) ccw projected
  line L2 (89.9, 47.9) -> (10.5, 47.9) projected
  arc A764 (10.5, 47.9) -> (10, 47.4) centre (10.5, 47.4) ccw projected
  line L3 (10, 47.4) -> (10, 36.65) projected
  arc A765 (9.5, 36.15) -> (10, 36.65) centre (9.5, 36.65) ccw projected
  line L4 (9.5, 36.15) -> (0.5, 36.15) projected
  line L5 (0, 35.65) -> (0.5, 36.15) projected
  line L6 (0, 35.65) -> (0, 25.45) projected
  line L7 (0.5, 24.95) -> (0, 25.45) projected
  line L8 (0.5, 24.95) -> (8.4, 24.95) projected
  arc A766 (8.4, 23.05) -> (8.4, 24.95) centre (8.4, 24) ccw projected
  line L9 (8.4, 23.05) -> (0.5, 23.05) projected
  line L10 (0, 22.55) -> (0.5, 23.05) projected
  line L11 (0, 22.55) -> (0, -14.65) projected
  line L12 (0.5, -15.15) -> (0, -14.65) projected
  line L13 (0.5, -15.15) -> (10, -15.15) projected
  arc A767 (10, -18.65) -> (10, -15.15) centre (10, -16.9) ccw projected
  line L14 (10, -18.65) -> (2.5, -18.65) projected
  arc A768 (2.5, -18.65) -> (2, -19.15) centre (2.5, -19.15) ccw projected
  line L15 (2, -19.15) -> (2, -47.4) projected
  arc A769 (2, -47.4) -> (2.5, -47.9) centre (2.5, -47.4) ccw projected
  line L16 (2.5, -47.9) -> (89.9, -47.9) projected
  arc A770 (89.9, -47.9) -> (90.4, -47.4) centre (89.9, -47.4) ccw projected
  line L17 (90.4, -47.4) -> (90.4, -4) projected
  arc A771 (90.4, -4) -> (89.4, -3) centre (89.4, -4) ccw projected
  line L18 (89.4, -3) -> (75.9, -3) projected
  arc A772 (74.9, -2) -> (75.9, -3) centre (75.9, -2) ccw projected
  line L19 (74.9, -2) -> (74.9, 2) projected
  arc A773 (75.9, 3) -> (74.9, 2) centre (75.9, 2) ccw projected
  line L20 (75.9, 3) -> (89.4, 3) projected
  arc A774 (89.4, 3) -> (90.4, 4) centre (89.4, 4) ccw projected
  line L21 (90.4, 4) -> (90.4, 34) projected
  point P0 (0, 0)
  point P1 (1.5, -42.9)
  point P2 (9.5, 37.9)
  point P3 (9.5, 38.9)
  point P4 (1.5, -41.9)
  point P5 (9.5, 39.9)
  point P6 (1.5, -40.9)
  point P7 (9.5, 40.9)
  point P8 (1.5, -39.9)
  point P9 (9.5, 41.9)
  point P10 (1.5, -38.9)
  point P11 (9.5, 42.9)
  point P12 (1.5, -37.9)
  point P13 (9.5, 43.9)
  point P14 (1.5, -36.9)
  point P15 (8.5, 37.9)
  point P16 (0.5, -42.9)
  point P17 (8.5, 38.9)
  point P18 (0.5, -41.9)
  point P19 (8.5, 39.9)
  point P20 (0.5, -40.9)
  point P21 (8.5, 40.9)
  point P22 (0.5, -39.9)
  point P23 (8.5, 41.9)
  point P24 (0.5, -38.9)
  point P25 (8.5, 42.9)
  point P26 (0.5, -37.9)
  point P27 (8.5, 43.9)
  point P28 (0.5, -36.9)
  point P29 (7.5, 37.9)
  point P30 (-0.5, -42.9)
  point P31 (7.5, 38.9)
  point P32 (-0.5, -41.9)
  point P33 (7.5, 39.9)
  point P34 (-0.5, -40.9)
  point P35 (7.5, 40.9)
  point P36 (-0.5, -39.9)
  point P37 (7.5, 41.9)
  point P38 (-0.5, -38.9)
  point P39 (7.5, 42.9)
  point P40 (-0.5, -37.9)
  point P41 (7.5, 43.9)
  point P42 (-0.5, -36.9)
  point P43 (6.5, 37.9)
  point P44 (-1.5, -42.9)
  point P45 (6.5, 38.9)
  point P46 (-1.5, -41.9)
  point P47 (6.5, 39.9)
  point P48 (-1.5, -40.9)
  point P49 (6.5, 40.9)
  point P50 (-1.5, -39.9)
  point P51 (6.5, 41.9)
  point P52 (-1.5, -38.9)
  point P53 (6.5, 42.9)
  point P54 (-1.5, -37.9)
  point P55 (6.5, 43.9)
  point P56 (-1.5, -36.9)
  dimension "d159" = 0.5
  dimension "d161" = 5
  dimension "d162" = 0.5
  dimension "d163" = 10
  dimension "d166" = 1
  dimension "d169" = 1
  constraints: 1 horizontal, 1 vertical, 54 other
  measures "d159" distance from line of L15 point (1.5, -42.9)
  measures "d161" distance from line of point (1.5, -42.9) L16
  measures "d162" distance from line of point (9.5, 37.9) L3
  measures "d163" distance from line of point (9.5, 37.9) L2
  measures "d166" distance of point (9.5, 37.9) point (9.5, 38.9)
  measures "d169" distance of point (9.5, 37.9) point (8.5, 37.9)
ref_plane "Work Plane1" through (16, 0, 0) normal (1, 0, 0) x (0, 1, 0)
sketch "Sketch19" plane through (16, 0, 0) normal (1, 0, 0) x (0, 1, 0)
  line L0 (-4, -0.8) -> (-4, 0.8) projected
  line L1 (-47.4, 0.8) -> (-4, 0.8) projected
  line L2 (-47.4, -0.8) -> (-47.4, 0.8) projected
  line L3 (-4, -0.8) -> (-47.4, -0.8) projected
  point P0 (0, 0)
  point P1 (-42.9, 1.8)
  point P2 (37.9, 1.8)
  point P3 (-42.9, 0)
  point P4 (37.9, 0)
  point P5 (-42.9, 2.8)
  point P6 (37.9, 2.8)
  point P7 (-41.9, 1.8)
  point P8 (38.9, 1.8)
  point P9 (-41.9, 2.8)
  point P10 (38.9, 2.8)
  point P11 (-40.9, 1.8)
  point P12 (39.9, 1.8)
  point P13 (-40.9, 2.8)
  point P14 (39.9, 2.8)
  point P15 (-39.9, 1.8)
  point P16 (40.9, 1.8)
  point P17 (-39.9, 2.8)
  point P18 (40.9, 2.8)
  point P19 (-38.9, 1.8)
  point P20 (41.9, 1.8)
  point P21 (-38.9, 2.8)
  point P22 (41.9, 2.8)
  point P23 (-37.9, 1.8)
  point P24 (42.9, 1.8)
  point P25 (-37.9, 2.8)
  point P26 (42.9, 2.8)
  point P27 (-36.9, 1.8)
  point P28 (43.9, 1.8)
  point P29 (-36.9, 2.8)
  point P30 (43.9, 2.8)
  point P31 (-42.9, 3.8)
  point P32 (37.9, 3.8)
  point P33 (-41.9, 3.8)
  point P34 (38.9, 3.8)
  point P35 (-40.9, 3.8)
  point P36 (39.9, 3.8)
  point P37 (-39.9, 3.8)
  point P38 (40.9, 3.8)
  point P39 (-38.9, 3.8)
  point P40 (41.9, 3.8)
  point P41 (-37.9, 3.8)
  point P42 (42.9, 3.8)
  point P43 (-36.9, 3.8)
  point P44 (43.9, 3.8)
  point P45 (-42.9, 4.8)
  point P46 (37.9, 4.8)
  point P47 (-41.9, 4.8)
  point P48 (38.9, 4.8)
  point P49 (-40.9, 4.8)
  point P50 (39.9, 4.8)
  point P51 (-39.9, 4.8)
  point P52 (40.9, 4.8)
  point P53 (-38.9, 4.8)
  point P54 (41.9, 4.8)
  point P55 (-37.9, 4.8)
  point P56 (42.9, 4.8)
  point P57 (-36.9, 4.8)
  point P58 (43.9, 4.8)
  point P59 (-42.9, 5.8)
  point P60 (37.9, 5.8)
  point P61 (-41.9, 5.8)
  point P62 (38.9, 5.8)
  point P63 (-40.9, 5.8)
  point P64 (39.9, 5.8)
  point P65 (-39.9, 5.8)
  point P66 (40.9, 5.8)
  point P67 (-38.9, 5.8)
  point P68 (41.9, 5.8)
  point P69 (-37.9, 5.8)
  point P70 (42.9, 5.8)
  point P71 (-36.9, 5.8)
  point P72 (43.9, 5.8)
  point P73 (-42.9, 6.8)
  point P74 (37.9, 6.8)
  point P75 (-41.9, 6.8)
  point P76 (38.9, 6.8)
  point P77 (-40.9, 6.8)
  point P78 (39.9, 6.8)
  point P79 (-39.9, 6.8)
  point P80 (40.9, 6.8)
  point P81 (-38.9, 6.8)
  point P82 (41.9, 6.8)
  point P83 (-37.9, 6.8)
  point P84 (42.9, 6.8)
  point P85 (-36.9, 6.8)
  point P86 (43.9, 6.8)
  point P87 (-42.9, 7.8)
  point P88 (37.9, 7.8)
  point P89 (-41.9, 7.8)
  point P90 (38.9, 7.8)
  point P91 (-40.9, 7.8)
  point P92 (39.9, 7.8)
  point P93 (-39.9, 7.8)
  point P94 (40.9, 7.8)
  point P95 (-38.9, 7.8)
  point P96 (41.9, 7.8)
  point P97 (-37.9, 7.8)
  point P98 (42.9, 7.8)
  point P99 (-36.9, 7.8)
  point P100 (43.9, 7.8)
  dimension "d175" = 1
  dimension "d178" = 1
  dimension "d181" = 1
  constraints: 2 vertical alignment, 1 horizontal, 1 horizontal alignment, 1 vertical, 96 other
  measures "d175" distance of point (-42.9, 1.8) point (-42.9, 2.8)
  measures "d178" distance of point (-42.9, 1.8) point (-41.9, 1.8)
  measures "d181" distance from line of L1 point (-42.9, 1.8)
ref_plane "Work Plane2" through (41, 0, 0) normal (1, 0, 0) x (0, 1, 0)
sketch "Sketch20" plane through (41, 0, 0) normal (1, 0, 0) x (0, 1, 0)
  point P0 (0, 0)
  point P1 (-42.9, 1.8)
  point P2 (-42.9, 2.8)
  point P3 (-41.9, 2.8)
  point P4 (-41.9, 1.8)
  point P5 (-40.9, 1.8)
  point P6 (-40.9, 2.8)
  point P7 (-39.9, 2.8)
  point P8 (-39.9, 1.8)
  point P9 (-38.9, 1.8)
  point P10 (-38.9, 2.8)
  point P11 (-37.9, 1.8)
  point P12 (-37.9, 2.8)
  point P13 (-36.9, 2.8)
  point P14 (-36.9, 1.8)
  point P15 (37.9, 1.8)
  point P16 (38.9, 1.8)
  point P17 (39.9, 1.8)
  point P18 (40.9, 1.8)
  point P19 (41.9, 1.8)
  point P20 (42.9, 1.8)
  point P21 (43.9, 1.8)
  point P22 (43.9, 2.8)
  point P23 (42.9, 2.8)
  point P24 (41.9, 2.8)
  point P25 (40.9, 2.8)
  point P26 (39.9, 2.8)
  point P27 (38.9, 2.8)
  point P28 (37.9, 2.8)
  point P29 (-42.9, 3.8)
  point P30 (-41.9, 3.8)
  point P31 (-40.9, 3.8)
  point P32 (-39.9, 3.8)
ref_plane "Work Plane3" through (4, 0, 0) normal (1, 0, 0) x (0, 1, 0)
sketch "Sketch21" plane through (4, 0, 0) normal (1, 0, 0) x (0, 1, 0)
  point P0 (0, 0)
  point P1 (-42.9, 3.8)
  point P2 (-41.9, 3.8)
  point P3 (-40.9, 3.8)
  point P4 (-39.9, 3.8)
  point P5 (-38.9, 3.8)
  point P6 (-37.9, 3.8)
  point P7 (-36.9, 3.8)
  point P8 (-36.9, 4.8)
  point P9 (-37.9, 4.8)
  point P10 (-38.9, 4.8)
  point P11 (-39.9, 4.8)
  point P12 (-40.9, 4.8)
  point P13 (-41.9, 4.8)
  point P14 (-42.9, 4.8)
equation "\"d23\" = d22"
equation "\"d25\" = d22"
equation "\"d42\" = d39"
equation "\"d45\" = d39"
body "Solid1"
